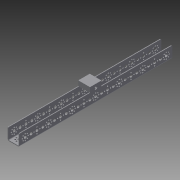
# Autodesk Inventor part: DropCenter Robot Part
Saved by Autodesk Inventor 2015 (Build 190159000, 159)
## iProperties
Created: 2012-09-30
Part Number: DropCenter Robot Part
Material: Generic
Document SubType Name: Sheet Metal
Designer: Nemo
Density: 1 g/cm^3
Sheet Metal Rule: Default_mm
Appearance: Default
Author: Nemo
Autodesk Inventor part; units mm, degrees
ref_plane "YZ Plane" through (0, 0, 0) normal (1, 0, 0) x (0, 1, 0)
ref_plane "XZ Plane" through (0, 0, 0) normal (0, 1, 0) x (-1, 0, 0)
ref_plane "XY Plane" through (0, 0, 0) normal (0, 0, 1) x (1, 0, 0)
sketch "Sketch1" plane through (0, 0, 0) normal (0, 0, 1) x (1, 0, 0)
  line L0 (-16, 208) -> (16, 208)
  line L1 (16, 208) -> (16, -208)
  line L2 (16, -208) -> (-16, -208)
  line L3 (-16, -208) -> (-16, 208)
  line L4 (-16, 0) -> (16, 0) construction
  circle A0 centre (0, 160) radius 4
  circle A1 centre (0, 160) radius 8 construction
  circle A2 centre (0, 168) radius 1.85
  circle A3 centre (0, 152) radius 1.85
  circle A4 centre (-8, 160) radius 1.85
  circle A5 centre (8, 160) radius 1.85
  circle A6 centre (0, 176) radius 4
  circle A7 centre (0, 144) radius 4
  circle A8 centre (0, 192) radius 4
  circle A9 centre (0, 192) radius 8 construction
  circle A10 centre (0, 200) radius 1.85
  circle A11 centre (-5.6569, 197.6569) radius 1.85
  circle A12 centre (-8, 192) radius 1.85
  circle A13 centre (-5.6569, 186.3431) radius 1.85
  circle A14 centre (0, 184) radius 1.85
  circle A15 centre (5.6569, 186.3431) radius 1.85
  circle A16 centre (8, 192) radius 1.85
  circle A17 centre (5.6569, 197.6569) radius 1.85
  circle A18 centre (0, 128) radius 4
  circle A19 centre (0, 128) radius 8 construction
  circle A20 centre (0, 136) radius 1.85
  circle A21 centre (-5.6569, 133.6569) radius 1.85
  circle A22 centre (-8, 128) radius 1.85
  circle A23 centre (-5.6569, 122.3431) radius 1.85
  circle A24 centre (0, 120) radius 1.85
  circle A25 centre (5.6569, 122.3431) radius 1.85
  circle A26 centre (8, 128) radius 1.85
  circle A27 centre (5.6569, 133.6569) radius 1.85
  circle A28 centre (0, 96) radius 4
  circle A29 centre (0, 96) radius 8 construction
  circle A30 centre (0, 104) radius 1.85
  circle A31 centre (0, 88) radius 1.85
  circle A32 centre (-8, 96) radius 1.85
  circle A33 centre (8, 96) radius 1.85
  circle A34 centre (0, 112) radius 4
  circle A35 centre (0, 80) radius 4
  circle A36 centre (0, 64) radius 4
  circle A37 centre (0, 64) radius 8 construction
  circle A38 centre (0, 72) radius 1.85
  circle A39 centre (-5.6569, 69.6569) radius 1.85
  circle A40 centre (-8, 64) radius 1.85
  circle A41 centre (-5.6569, 58.3431) radius 1.85
  circle A42 centre (0, 56) radius 1.85
  circle A43 centre (5.6569, 58.3431) radius 1.85
  circle A44 centre (8, 64) radius 1.85
  circle A45 centre (5.6569, 69.6569) radius 1.85
  circle A46 centre (0, 32) radius 4
  circle A47 centre (0, 32) radius 8 construction
  circle A48 centre (0, 40) radius 1.85
  circle A49 centre (0, 24) radius 1.85
  circle A50 centre (-8, 32) radius 1.85
  circle A51 centre (8, 32) radius 1.85
  circle A52 centre (0, 48) radius 4
  circle A53 centre (0, 16) radius 4
  circle A54 centre (0, 0) radius 4
  circle A55 centre (0, 0) radius 8 construction
  circle A56 centre (0, 8) radius 1.85
  circle A57 centre (-5.6569, 5.6569) radius 1.85
  circle A58 centre (-8, 0) radius 1.85
  circle A59 centre (-5.6569, -5.6569) radius 1.85
  circle A60 centre (0, -8) radius 1.85
  circle A61 centre (5.6569, -5.6569) radius 1.85
  circle A62 centre (8, 0) radius 1.85
  circle A63 centre (5.6569, 5.6569) radius 1.85
  circle A64 centre (0, -160) radius 4
  circle A65 centre (0, -160) radius 8 construction
  circle A66 centre (0, -168) radius 1.85
  circle A67 centre (0, -152) radius 1.85
  circle A68 centre (-8, -160) radius 1.85
  circle A69 centre (8, -160) radius 1.85
  circle A70 centre (0, -176) radius 4
  circle A71 centre (0, -144) radius 4
  circle A72 centre (0, -192) radius 4
  circle A73 centre (0, -192) radius 8 construction
  circle A74 centre (0, -200) radius 1.85
  circle A75 centre (-5.6569, -197.6569) radius 1.85
  circle A76 centre (-8, -192) radius 1.85
  circle A77 centre (-5.6569, -186.3431) radius 1.85
  circle A78 centre (0, -184) radius 1.85
  circle A79 centre (5.6569, -186.3431) radius 1.85
  circle A80 centre (8, -192) radius 1.85
  circle A81 centre (5.6569, -197.6569) radius 1.85
  circle A82 centre (0, -128) radius 4
  circle A83 centre (0, -128) radius 8 construction
  circle A84 centre (0, -136) radius 1.85
  circle A85 centre (-5.6569, -133.6569) radius 1.85
  circle A86 centre (-8, -128) radius 1.85
  circle A87 centre (-5.6569, -122.3431) radius 1.85
  circle A88 centre (0, -120) radius 1.85
  circle A89 centre (5.6569, -122.3431) radius 1.85
  circle A90 centre (8, -128) radius 1.85
  circle A91 centre (5.6569, -133.6569) radius 1.85
  circle A92 centre (0, -96) radius 4
  circle A93 centre (0, -96) radius 8 construction
  circle A94 centre (0, -104) radius 1.85
  circle A95 centre (0, -88) radius 1.85
  circle A96 centre (-8, -96) radius 1.85
  circle A97 centre (8, -96) radius 1.85
  circle A98 centre (0, -112) radius 4
  circle A99 centre (0, -80) radius 4
  circle A100 centre (0, -64) radius 4
  circle A101 centre (0, -64) radius 8 construction
  circle A102 centre (0, -72) radius 1.85
  circle A103 centre (-5.6569, -69.6569) radius 1.85
  circle A104 centre (-8, -64) radius 1.85
  circle A105 centre (-5.6569, -58.3431) radius 1.85
  circle A106 centre (0, -56) radius 1.85
  circle A107 centre (5.6569, -58.3431) radius 1.85
  circle A108 centre (8, -64) radius 1.85
  circle A109 centre (5.6569, -69.6569) radius 1.85
  circle A110 centre (0, -32) radius 4
  circle A111 centre (0, -32) radius 8 construction
  circle A112 centre (0, -40) radius 1.85
  circle A113 centre (0, -24) radius 1.85
  circle A114 centre (-8, -32) radius 1.85
  circle A115 centre (8, -32) radius 1.85
  circle A116 centre (0, -48) radius 4
  circle A117 centre (0, -16) radius 4
  point P0 (0, 208)
  dimension "d20" = 16
  dimension "d21" = 16
  dimension "d22" = 16
  dimension "d23" = 16
  dimension "d26" = 16
  dimension "d0" = 32
  dimension "d1" = 416
  dimension "d25" = 16
  measures "d0" distance of L1.end L2.end
  measures "d1" distance of L0.end L1.end
extrude "Plate1" add sketch "Sketch1" along normal blind 2
sketch "Sketch2" plane through (-14, -208, 0) normal (-1, 0, 0) x (0, -1, 0)
  line L0 (-416, 0) -> (0, 0)
  line L1 (0, 0) -> (0, 32)
  line L2 (0, 32) -> (-416, 32)
  line L3 (-416, 32) -> (-416, 0)
  constraints: 6 end point, 1 horizontal, 1 perpendicular, 1 vertical
edge flange "Flange1" height 32 angle 90 thickness 2 bend radius 2 thickness toward (-1, 0, 0) relief tear relief width 2 relief depth 1 corner gap 2 corner form 0 edges at (-16, 0, 2) (16, 0, 2) wall of the first edge with corners at (-14, 208, 0) (-14, -208, 0) (-14, -208, 32) (-14, 208, 32)
bend "Bend1"
corner "Corner1"
sketch "Hole Pattern 4" plane through (0, 0, 0) normal (0, 0, 1) x (1, 0, 0)
  circle A0 centre (-145.7144, 104.3642) radius 4
  circle A1 centre (-145.7144, 104.3642) radius 8 construction
  circle A2 centre (-145.7144, 112.3642) radius 1.85
  circle A3 centre (-145.7144, 96.3642) radius 1.85
  circle A4 centre (-153.7144, 104.3642) radius 1.85
  circle A5 centre (-137.7144, 104.3642) radius 1.85
  circle A6 centre (-145.7144, 120.3642) radius 4
  circle A7 centre (-145.7144, 88.3642) radius 4
  point P0 (-145.7144, 107.7928)
  dimension "d3" = 16
  dimension "d4" = 3.7
  dimension "d8" = 16
  dimension "d9" = 16
  dimension "d10" = 8
  measures "d3" diameter of A1
  measures "d4" diameter of A2
  measures "d8" distance of A6.centre A0.centre
  measures "d9" distance of A7.centre A0.centre
  measures "d10" diameter of A0
sketch "Hole Pattern 8" plane through (0, 0, 0) normal (0, 0, 1) x (1, 0, 0)
  circle A0 centre (-147.7869, 106.9769) radius 4
  circle A1 centre (-147.7869, 106.9769) radius 8 construction
  circle A2 centre (-147.7869, 114.9769) radius 1.85
  circle A3 centre (-153.4437, 112.6338) radius 1.85
  circle A4 centre (-155.7869, 106.9769) radius 1.85
  circle A5 centre (-153.4437, 101.3201) radius 1.85
  circle A6 centre (-147.7869, 98.9769) radius 1.85
  circle A7 centre (-142.13, 101.3201) radius 1.85
  circle A8 centre (-139.7869, 106.9769) radius 1.85
  circle A9 centre (-142.13, 112.6338) radius 1.85
  point P0 (-145.7144, 107.7928)
  dimension "d6" = 16
  dimension "d13" = 3.7
  dimension "d14" = 8
  dimension "d17" = 360
  measures "d13" diameter of A2
  measures "d14" diameter of A0
sketch "416 mm hole pattern" plane through (0, 0, 0) normal (0, 0, 1) x (1, 0, 0)
  line L0 (-16, 0) -> (16, 0) construction
  circle A0 centre (0, 160) radius 4
  circle A1 centre (0, 160) radius 8 construction
  circle A2 centre (0, 168) radius 1.85
  circle A3 centre (0, 152) radius 1.85
  circle A4 centre (-8, 160) radius 1.85
  circle A5 centre (8, 160) radius 1.85
  circle A6 centre (0, 176) radius 4
  circle A7 centre (0, 144) radius 4
  circle A8 centre (0, 192) radius 4
  circle A9 centre (0, 192) radius 8 construction
  circle A10 centre (0, 200) radius 1.85
  circle A11 centre (-5.6569, 197.6569) radius 1.85
  circle A12 centre (-8, 192) radius 1.85
  circle A13 centre (-5.6569, 186.3431) radius 1.85
  circle A14 centre (0, 184) radius 1.85
  circle A15 centre (5.6569, 186.3431) radius 1.85
  circle A16 centre (8, 192) radius 1.85
  circle A17 centre (5.6569, 197.6569) radius 1.85
  circle A18 centre (0, 128) radius 4
  circle A19 centre (0, 128) radius 8 construction
  circle A20 centre (0, 136) radius 1.85
  circle A21 centre (-5.6569, 133.6569) radius 1.85
  circle A22 centre (-8, 128) radius 1.85
  circle A23 centre (-5.6569, 122.3431) radius 1.85
  circle A24 centre (0, 120) radius 1.85
  circle A25 centre (5.6569, 122.3431) radius 1.85
  circle A26 centre (8, 128) radius 1.85
  circle A27 centre (5.6569, 133.6569) radius 1.85
  circle A28 centre (0, 96) radius 4
  circle A29 centre (0, 96) radius 8 construction
  circle A30 centre (0, 104) radius 1.85
  circle A31 centre (0, 88) radius 1.85
  circle A32 centre (-8, 96) radius 1.85
  circle A33 centre (8, 96) radius 1.85
  circle A34 centre (0, 112) radius 4
  circle A35 centre (0, 80) radius 4
  circle A36 centre (0, 64) radius 4
  circle A37 centre (0, 64) radius 8 construction
  circle A38 centre (0, 72) radius 1.85
  circle A39 centre (-5.6569, 69.6569) radius 1.85
  circle A40 centre (-8, 64) radius 1.85
  circle A41 centre (-5.6569, 58.3431) radius 1.85
  circle A42 centre (0, 56) radius 1.85
  circle A43 centre (5.6569, 58.3431) radius 1.85
  circle A44 centre (8, 64) radius 1.85
  circle A45 centre (5.6569, 69.6569) radius 1.85
  circle A46 centre (0, 32) radius 4
  circle A47 centre (0, 32) radius 8 construction
  circle A48 centre (0, 40) radius 1.85
  circle A49 centre (0, 24) radius 1.85
  circle A50 centre (-8, 32) radius 1.85
  circle A51 centre (8, 32) radius 1.85
  circle A52 centre (0, 48) radius 4
  circle A53 centre (0, 16) radius 4
  circle A54 centre (0, 0) radius 4
  circle A55 centre (0, 0) radius 8 construction
  circle A56 centre (0, 8) radius 1.85
  circle A57 centre (-5.6569, 5.6569) radius 1.85
  circle A58 centre (-8, 0) radius 1.85
  circle A59 centre (-5.6569, -5.6569) radius 1.85
  circle A60 centre (0, -8) radius 1.85
  circle A61 centre (5.6569, -5.6569) radius 1.85
  circle A62 centre (8, 0) radius 1.85
  circle A63 centre (5.6569, 5.6569) radius 1.85
  circle A64 centre (0, -160) radius 4
  circle A65 centre (0, -160) radius 8 construction
  circle A66 centre (0, -168) radius 1.85
  circle A67 centre (0, -152) radius 1.85
  circle A68 centre (-8, -160) radius 1.85
  circle A69 centre (8, -160) radius 1.85
  circle A70 centre (0, -176) radius 4
  circle A71 centre (0, -144) radius 4
  circle A72 centre (0, -192) radius 4
  circle A73 centre (0, -192) radius 8 construction
  circle A74 centre (0, -200) radius 1.85
  circle A75 centre (-5.6569, -197.6569) radius 1.85
  circle A76 centre (-8, -192) radius 1.85
  circle A77 centre (-5.6569, -186.3431) radius 1.85
  circle A78 centre (0, -184) radius 1.85
  circle A79 centre (5.6569, -186.3431) radius 1.85
  circle A80 centre (8, -192) radius 1.85
  circle A81 centre (5.6569, -197.6569) radius 1.85
  circle A82 centre (0, -128) radius 4
  circle A83 centre (0, -128) radius 8 construction
  circle A84 centre (0, -136) radius 1.85
  circle A85 centre (-5.6569, -133.6569) radius 1.85
  circle A86 centre (-8, -128) radius 1.85
  circle A87 centre (-5.6569, -122.3431) radius 1.85
  circle A88 centre (0, -120) radius 1.85
  circle A89 centre (5.6569, -122.3431) radius 1.85
  circle A90 centre (8, -128) radius 1.85
  circle A91 centre (5.6569, -133.6569) radius 1.85
  circle A92 centre (0, -96) radius 4
  circle A93 centre (0, -96) radius 8 construction
  circle A94 centre (0, -104) radius 1.85
  circle A95 centre (0, -88) radius 1.85
  circle A96 centre (-8, -96) radius 1.85
  circle A97 centre (8, -96) radius 1.85
  circle A98 centre (0, -112) radius 4
  circle A99 centre (0, -80) radius 4
  circle A100 centre (0, -64) radius 4
  circle A101 centre (0, -64) radius 8 construction
  circle A102 centre (0, -72) radius 1.85
  circle A103 centre (-5.6569, -69.6569) radius 1.85
  circle A104 centre (-8, -64) radius 1.85
  circle A105 centre (-5.6569, -58.3431) radius 1.85
  circle A106 centre (0, -56) radius 1.85
  circle A107 centre (5.6569, -58.3431) radius 1.85
  circle A108 centre (8, -64) radius 1.85
  circle A109 centre (5.6569, -69.6569) radius 1.85
  circle A110 centre (0, -32) radius 4
  circle A111 centre (0, -32) radius 8 construction
  circle A112 centre (0, -40) radius 1.85
  circle A113 centre (0, -24) radius 1.85
  circle A114 centre (-8, -32) radius 1.85
  circle A115 centre (8, -32) radius 1.85
  circle A116 centre (0, -48) radius 4
  circle A117 centre (0, -16) radius 4
  point P0 (0.806, 0.0453)
  dimension "d38" = 16
  dimension "d39" = 16
  dimension "d40" = 16
  dimension "d41" = 16
  dimension "d43" = 16
  dimension "d42" = 16
sketch "Sketch3" plane through (-16, -208, 32) normal (-1, 0, 0) x (0, 0, 1)
  line L0 (-32, 0) -> (-32, 416) construction
  line L1 (0, 416) -> (0, 0) construction
  line L2 (-32, 416) -> (0, 416) construction
  line L3 (-32, 0) -> (0, 0) construction
  line L4 (-32, 208) -> (0, 208) construction
  circle A0 centre (-16, 368) radius 4
  circle A1 centre (-16, 368) radius 8 construction
  circle A2 centre (-16, 376) radius 1.85
  circle A3 centre (-16, 360) radius 1.85
  circle A4 centre (-24, 368) radius 1.85
  circle A5 centre (-8, 368) radius 1.85
  circle A6 centre (-16, 384) radius 4
  circle A7 centre (-16, 352) radius 4
  circle A8 centre (-16, 400) radius 4
  circle A9 centre (-16, 400) radius 8 construction
  circle A10 centre (-16, 408) radius 1.85
  circle A11 centre (-21.6569, 405.6569) radius 1.85
  circle A12 centre (-24, 400) radius 1.85
  circle A13 centre (-21.6569, 394.3431) radius 1.85
  circle A14 centre (-16, 392) radius 1.85
  circle A15 centre (-10.3431, 394.3431) radius 1.85
  circle A16 centre (-8, 400) radius 1.85
  circle A17 centre (-10.3431, 405.6569) radius 1.85
  circle A18 centre (-16, 336) radius 4
  circle A19 centre (-16, 336) radius 8 construction
  circle A20 centre (-16, 344) radius 1.85
  circle A21 centre (-21.6569, 341.6569) radius 1.85
  circle A22 centre (-24, 336) radius 1.85
  circle A23 centre (-21.6569, 330.3431) radius 1.85
  circle A24 centre (-16, 328) radius 1.85
  circle A25 centre (-10.3431, 330.3431) radius 1.85
  circle A26 centre (-8, 336) radius 1.85
  circle A27 centre (-10.3431, 341.6569) radius 1.85
  circle A28 centre (-16, 304) radius 4
  circle A29 centre (-16, 304) radius 8 construction
  circle A30 centre (-16, 312) radius 1.85
  circle A31 centre (-16, 296) radius 1.85
  circle A32 centre (-24, 304) radius 1.85
  circle A33 centre (-8, 304) radius 1.85
  circle A34 centre (-16, 320) radius 4
  circle A35 centre (-16, 288) radius 4
  circle A36 centre (-16, 272) radius 4
  circle A37 centre (-16, 272) radius 8 construction
  circle A38 centre (-16, 280) radius 1.85
  circle A39 centre (-21.6569, 277.6569) radius 1.85
  circle A40 centre (-24, 272) radius 1.85
  circle A41 centre (-21.6569, 266.3431) radius 1.85
  circle A42 centre (-16, 264) radius 1.85
  circle A43 centre (-10.3431, 266.3431) radius 1.85
  circle A44 centre (-8, 272) radius 1.85
  circle A45 centre (-10.3431, 277.6569) radius 1.85
  circle A46 centre (-16, 240) radius 4
  circle A47 centre (-16, 240) radius 8 construction
  circle A48 centre (-16, 248) radius 1.85
  circle A49 centre (-16, 232) radius 1.85
  circle A50 centre (-24, 240) radius 1.85
  circle A51 centre (-8, 240) radius 1.85
  circle A52 centre (-16, 256) radius 4
  circle A53 centre (-16, 224) radius 4
  circle A54 centre (-16, 208) radius 4
  circle A55 centre (-16, 208) radius 8 construction
  circle A56 centre (-16, 216) radius 1.85
  circle A57 centre (-21.6569, 213.6569) radius 1.85
  circle A58 centre (-24, 208) radius 1.85
  circle A59 centre (-21.6569, 202.3431) radius 1.85
  circle A60 centre (-16, 200) radius 1.85
  circle A61 centre (-10.3431, 202.3431) radius 1.85
  circle A62 centre (-8, 208) radius 1.85
  circle A63 centre (-10.3431, 213.6569) radius 1.85
  circle A64 centre (-16, 48) radius 4
  circle A65 centre (-16, 48) radius 8 construction
  circle A66 centre (-16, 40) radius 1.85
  circle A67 centre (-16, 56) radius 1.85
  circle A68 centre (-24, 48) radius 1.85
  circle A69 centre (-8, 48) radius 1.85
  circle A70 centre (-16, 32) radius 4
  circle A71 centre (-16, 64) radius 4
  circle A72 centre (-16, 16) radius 4
  circle A73 centre (-16, 16) radius 8 construction
  circle A74 centre (-16, 8) radius 1.85
  circle A75 centre (-21.6569, 10.3431) radius 1.85
  circle A76 centre (-24, 16) radius 1.85
  circle A77 centre (-21.6569, 21.6569) radius 1.85
  circle A78 centre (-16, 24) radius 1.85
  circle A79 centre (-10.3431, 21.6569) radius 1.85
  circle A80 centre (-8, 16) radius 1.85
  circle A81 centre (-10.3431, 10.3431) radius 1.85
  circle A82 centre (-16, 80) radius 4
  circle A83 centre (-16, 80) radius 8 construction
  circle A84 centre (-16, 72) radius 1.85
  circle A85 centre (-21.6569, 74.3431) radius 1.85
  circle A86 centre (-24, 80) radius 1.85
  circle A87 centre (-21.6569, 85.6569) radius 1.85
  circle A88 centre (-16, 88) radius 1.85
  circle A89 centre (-10.3431, 85.6569) radius 1.85
  circle A90 centre (-8, 80) radius 1.85
  circle A91 centre (-10.3431, 74.3431) radius 1.85
  circle A92 centre (-16, 112) radius 4
  circle A93 centre (-16, 112) radius 8 construction
  circle A94 centre (-16, 104) radius 1.85
  circle A95 centre (-16, 120) radius 1.85
  circle A96 centre (-24, 112) radius 1.85
  circle A97 centre (-8, 112) radius 1.85
  circle A98 centre (-16, 96) radius 4
  circle A99 centre (-16, 128) radius 4
  circle A100 centre (-16, 144) radius 4
  circle A101 centre (-16, 144) radius 8 construction
  circle A102 centre (-16, 136) radius 1.85
  circle A103 centre (-21.6569, 138.3431) radius 1.85
  circle A104 centre (-24, 144) radius 1.85
  circle A105 centre (-21.6569, 149.6569) radius 1.85
  circle A106 centre (-16, 152) radius 1.85
  circle A107 centre (-10.3431, 149.6569) radius 1.85
  circle A108 centre (-8, 144) radius 1.85
  circle A109 centre (-10.3431, 138.3431) radius 1.85
  circle A110 centre (-16, 176) radius 4
  circle A111 centre (-16, 176) radius 8 construction
  circle A112 centre (-16, 168) radius 1.85
  circle A113 centre (-16, 184) radius 1.85
  circle A114 centre (-24, 176) radius 1.85
  circle A115 centre (-8, 176) radius 1.85
  circle A116 centre (-16, 160) radius 4
  circle A117 centre (-16, 192) radius 4
  dimension "d45" = 16
  constraints: 4 end point, 1 midpoint, 1 parallel, 1 perpendicular, 1 other
extrude "Extrusion1" cut sketch "Sketch3" against normal through all
fillet "Fillet1" radius 2 4 edges at (-15, -208, 32) (15, -208, 32) (-15, 208, 32) (15, 208, 32)
sketch "Sketch4" plane through (-16, -208, 4) normal (-1, 0, 0) x (0, 0, 1)
  circle A0 centre (30.6551, 208) radius 4.8273
  line L0 (28, 2) -> (28, 414) projected
  line L1 (41.4884, 192) -> (28, 192)
  line L2 (28, 192) -> (28, 223.3008)
  line L3 (28, 223.3008) -> (41.4884, 223.3008)
  line L4 (41.4884, 223.3008) -> (41.4884, 192)
  point P0 (-4, 208)
  constraints: 8 end point, 2 parallel, 1 centre point, 1 horizontal, 1 perpendicular, 1 point on line
extrude "Extrusion2" add sketch "Sketch4" against normal blind 32 contours A0 L0 | A0 L0 L3 L4 L1 picked at (30.4483, 208.3813)
sketch "Sketch5" plane through (-16, -208, 4) normal (-1, 0, 0) x (0, 0, 1)
  circle A0 centre (12, 208) radius 4 projected
  line L0 (12, 208) -> (31.4748, 208)
  point P0 (-4, 208)
  constraints: 2 end point, 1 horizontal
hole "Hole1" at (-16, 0, 35.4748) direction (1, 0, 0) diameter 8 end through all
equation "\"d56\" = Thickness"
equation "\"d28\" = BendReliefWidth"
equation "\"d29\" = BendReliefDepth"
equation "\"d30\" = MinimumRemnant"
equation "\"d31\" = BendRadius"
equation "\"d34\" = BendRadius"
equation "\"d35\" = CornerReliefSize"
equation "\"d36\" = GapSize"
equation "\"d37\" = JacobiRadiusSize"
equation "\"BendRadius\" = Thickness"
equation "\"BendReliefWidth\" = Thickness"
equation "\"BendReliefDepth\" = 0.5 * Thickness"
equation "\"CornerReliefSize\" = 4 * Thickness"
equation "\"MinimumRemnant\" = 2 * Thickness"
equation "\"TransitionRadius\" = BendRadius"
equation "\"JacobiRadiusSize\" = BendRadius"
equation "\"GapSize\" = Thickness"
equation "\"d27\" = BendRadius"
equation "\"Thickness\" = 2"
body "Solid1"
